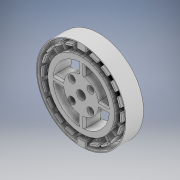
# Autodesk Inventor part: Kotač_v.2.0
Saved by Autodesk Inventor 2020 (Build 240168000, 168)
## iProperties
Created: 2020-03-09
Part Number: Kotač_v.2.0
Material: Generic
Document SubType Name: Modeling
Designer: Jadran Jelčić
Density: 1 g/cm^3
Appearance: Default
Author: Jadran Jelčić
Autodesk Inventor part; units mm, degrees
ref_plane "YZ Plane" through (0, 0, 0) normal (1, 0, 0) x (0, 1, 0)
ref_plane "XZ Plane" through (0, 0, 0) normal (0, 1, 0) x (-1, 0, 0)
ref_plane "XY Plane" through (0, 0, 0) normal (0, 0, 1) x (1, 0, 0)
sketch "Sketch1" plane through (0, 0, 0) normal (0, 0, 1) x (1, 0, 0)
  circle A0 centre (0, 0) radius 19
  circle A1 centre (0, 0) radius 10
  circle A2 centre (0, 0) radius 2.5
  line L0 (0, 0) -> (-75, 0)
  line L1 (0, 0) -> (-7.5, 0)
  circle A3 centre (-7.5, 0) radius 2
  circle A4 centre (0, -7.5) radius 2
  circle A5 centre (7.5, 0) radius 2
  circle A6 centre (0, 7.5) radius 2
  circle A7 centre (0, 0) radius 16
  line L2 (-9.8406, 1.7786) -> (-15.9008, 1.7786)
  line L3 (-9.8331, -1.8195) -> (-15.8962, -1.8195)
  line L4 (-1.7786, -9.8406) -> (-1.7786, -15.9008)
  line L5 (1.8195, -9.8331) -> (1.8195, -15.8962)
  line L6 (9.8406, -1.7786) -> (15.9008, -1.7786)
  line L7 (9.8331, 1.8195) -> (15.8962, 1.8195)
  line L8 (1.7786, 9.8406) -> (1.7786, 15.9008)
  line L9 (-1.8195, 9.8331) -> (-1.8195, 15.8962)
  line L10 (0, -7.5) -> (-7.5, 0)
  line L11 (0, 0) -> (-9.2351, -9.2351)
  line L12 (0, 0) -> (13.0604, 0) construction
  circle A8 centre (-5.3039, -5.3039) radius 2
  circle A9 centre (5.3039, -5.3039) radius 2
  circle A10 centre (5.3039, 5.3039) radius 2
  circle A11 centre (-5.3039, 5.3039) radius 2
  point P0 (-1.7786, -9.8406)
  point P1 (-1.7786, -15.9008)
  point P2 (1.8195, -15.8962)
  point P3 (1.8195, -9.8331)
  point P4 (9.8406, -1.7786)
  point P5 (15.8962, 1.8195)
  point P6 (9.8331, 1.8195)
  point P7 (1.7786, 9.8406)
  point P8 (-1.8195, 15.8962)
  point P9 (-1.8195, 9.8331)
  dimension "d0" = 38
  dimension "d1" = 20
  dimension "d2" = 5
  dimension "d5" = 4
  dimension "d8" = 360
  dimension "d12" = 360
  dimension "d23" = 32
  dimension "d31" = 135
  dimension "d32" = 4
  dimension "d35" = 360
  constraints: 26 end point, 12 centre point, 5 coincident, 4 point on circle, 2 horizontal, 2 parallel, 2 point on line, 1 equal length, 43 other
  measures "d0" diameter of A0
  measures "d1" diameter of A1
  measures "d2" diameter of A2
  measures "d5" diameter of A3
  measures "d23" diameter of A7
  measures "d31" angle of L11 L12
  measures "d32" diameter of A8
extrude "Extrusion1" add sketch "Sketch1" along normal blind 10 contours A0 | A1 L11 A8 A2 L0 A3 | A1 L7 A7 L6 | A1 L9 A7 L8 | L5 A7 L4 A1 | A1 L0 A7 L2 | A1 L0 A3 L10 L11 A8 | A1 L3 A7 L0 | A8 L11 | L11 A8 | L0 A2 L11 L10 A3 | A9 | A10 | A11
sketch "Sketch2" plane through (0, 0, 10) normal (0, 0, 1) x (1, 0, 0)
  circle A0 centre (0, 0) radius 2.5 projected
  circle A1 centre (0, 0) radius 19 projected
  line L0 (-19, 0) -> (-23, 0)
  line L1 (-23, 0) -> (-23, 0.991)
  line L2 (-23, 0.991) -> (-18.9741, 0.991)
  line L3 (-23, 0.991) -> (-23, 2.3883)
  line L4 (-23, 2.3883) -> (-22, 2.3883)
  line L5 (-22, 2.3883) -> (-22, 0.991)
  line L6 (-23, 0) -> (-23, -0.991)
  line L7 (-23, -0.991) -> (-18.9741, -0.991)
  line L8 (-23, -0.991) -> (-23, -2.3883)
  line L9 (-23, -2.3883) -> (-22, -2.3883)
  line L10 (-22, -2.3883) -> (-22, -0.991)
  point P0 (-18.9741, -0.991)
  dimension "d18" = 1
  dimension "d19" = 4
  constraints: 22 end point, 5 symmetric about line, 4 perpendicular, 2 point on circle, 2 point on line, 1 horizontal, 1 vertical
  measures "d18" distance between parallel lines of L5 L3
  measures "d19" distance from line of L0.start L1
extrude "Extrusion7" add sketch "Sketch2" against normal blind 10 contours A1 L0 L1 L2 | L7 L6 L0 A1 | L2 L3 L4 L5 | L10 L9 L8 L7
pattern_circular "Circular Pattern2" count 20 over 360 about axis through (0, 0, 0) along (0, 0, 1) of "Extrusion7"
sketch "Sketch4" plane through (0, 0, 10) normal (0, 0, 1) x (1, 0, 0)
  line L0 (0, 0) -> (-2.7237, 0)
  line L1 (2.3883, -22) -> (2.3883, -23) projected
  line L2 (2.3883, -23) -> (-2.3771, -23)
  line L3 (-2.3771, -23) -> (-2.3771, -25)
  line L4 (-2.3771, -25) -> (2.3883, -25)
  line L5 (2.3883, -25) -> (2.3883, -23)
  line L6 (2.3883, 22) -> (2.3883, 23)
  line L7 (2.3883, 23) -> (-2.3771, 23)
  line L8 (-2.3771, 23) -> (-2.3771, 25)
  line L9 (-2.3771, 25) -> (2.3883, 25)
  line L10 (2.3883, 25) -> (2.3883, 23)
  dimension "d52" = 2
  constraints: 20 end point, 5 symmetric about line, 2 horizontal, 2 parallel, 1 perpendicular
  measures "d52" distance of L3.end L2.end
extrude "Extrusion8" add sketch "Sketch4" against normal blind 1
sketch "Sketch5" plane through (0, 0, 10) normal (0, 0, 1) x (1, 0, 0)
  circle A0 centre (0, 0) radius 2.5 projected
  circle A1 centre (0, 0) radius 25
  circle A2 centre (0, 0) radius 25.5
  dimension "d27" = 50
  dimension "d28" = 51
  constraints: 2 centre point, 2 coincident
  measures "d27" diameter of A1
  measures "d28" diameter of A2
extrude "Extrusion4" add sketch "Sketch5" against normal blind 10 contours A2
sketch "Sketch8" plane through (0, 0, 10) normal (0, 0, 1) x (1, 0, 0)
  line L0 (-0.991, 18.9741) -> (-0.991, 22) projected
  line L1 (0.991, 22) -> (0.991, 18.9741) projected
  line L2 (-0.991, 22) -> (0.991, 22)
  line L3 (0.991, 22) -> (0.991, 18.9741)
  line L4 (0.991, 18.9741) -> (-0.991, 18.9741)
  line L5 (-0.991, 18.9741) -> (-0.991, 22)
  arc A0 (4.9208, 18.3517) -> (0.991, 18.9741) centre (0, 0) ccw projected
  line L6 (-6.8058, 17.7392) -> (-7.7409, 20.617)
  line L7 (-7.7409, 20.617) -> (-5.8559, 21.2295)
  line L8 (-5.8559, 21.2295) -> (-4.9208, 18.3517)
  line L9 (-4.9208, 18.3517) -> (-6.8058, 17.7392)
  line L10 (-11.9545, 14.7679) -> (-13.733, 17.2159)
  line L11 (-13.733, 17.2159) -> (-12.1295, 18.3809)
  line L12 (-12.1295, 18.3809) -> (-10.351, 15.9329)
  line L13 (-10.351, 15.9329) -> (-11.9545, 14.7679)
  line L14 (-15.9329, 10.351) -> (-18.3809, 12.1295)
  line L15 (-18.3809, 12.1295) -> (-17.2159, 13.733)
  line L16 (-17.2159, 13.733) -> (-14.7679, 11.9545)
  line L17 (-14.7679, 11.9545) -> (-15.9329, 10.351)
  line L18 (-18.3517, 4.9208) -> (-21.2295, 5.8559)
  line L19 (-21.2295, 5.8559) -> (-20.617, 7.7409)
  line L20 (-20.617, 7.7409) -> (-17.7392, 6.8058)
  line L21 (-17.7392, 6.8058) -> (-18.3517, 4.9208)
  line L22 (-18.9741, -0.991) -> (-22, -0.991)
  line L23 (-22, -0.991) -> (-22, 0.991)
  line L24 (-22, 0.991) -> (-18.9741, 0.991)
  line L25 (-18.9741, 0.991) -> (-18.9741, -0.991)
  line L26 (-17.7392, -6.8058) -> (-20.617, -7.7409)
  line L27 (-20.617, -7.7409) -> (-21.2295, -5.8559)
  line L28 (-21.2295, -5.8559) -> (-18.3517, -4.9208)
  line L29 (-18.3517, -4.9208) -> (-17.7392, -6.8058)
  line L30 (-14.7679, -11.9545) -> (-17.2159, -13.733)
  line L31 (-17.2159, -13.733) -> (-18.3809, -12.1295)
  line L32 (-18.3809, -12.1295) -> (-15.9329, -10.351)
  line L33 (-15.9329, -10.351) -> (-14.7679, -11.9545)
  line L34 (-10.351, -15.9329) -> (-12.1295, -18.3809)
  line L35 (-12.1295, -18.3809) -> (-13.733, -17.2159)
  line L36 (-13.733, -17.2159) -> (-11.9545, -14.7679)
  line L37 (-11.9545, -14.7679) -> (-10.351, -15.9329)
  line L38 (-4.9208, -18.3517) -> (-5.8559, -21.2295)
  line L39 (-5.8559, -21.2295) -> (-7.7409, -20.617)
  line L40 (-7.7409, -20.617) -> (-6.8058, -17.7392)
  line L41 (-6.8058, -17.7392) -> (-4.9208, -18.3517)
  line L42 (0.991, -18.9741) -> (0.991, -22)
  line L43 (0.991, -22) -> (-0.991, -22)
  line L44 (-0.991, -22) -> (-0.991, -18.9741)
  line L45 (-0.991, -18.9741) -> (0.991, -18.9741)
  line L46 (6.8058, -17.7392) -> (7.7409, -20.617)
  line L47 (7.7409, -20.617) -> (5.8559, -21.2295)
  line L48 (5.8559, -21.2295) -> (4.9208, -18.3517)
  line L49 (4.9208, -18.3517) -> (6.8058, -17.7392)
  line L50 (11.9545, -14.7679) -> (13.733, -17.2159)
  line L51 (13.733, -17.2159) -> (12.1295, -18.3809)
  line L52 (12.1295, -18.3809) -> (10.351, -15.9329)
  line L53 (10.351, -15.9329) -> (11.9545, -14.7679)
  line L54 (15.9329, -10.351) -> (18.3809, -12.1295)
  line L55 (18.3809, -12.1295) -> (17.2159, -13.733)
  line L56 (17.2159, -13.733) -> (14.7679, -11.9545)
  line L57 (14.7679, -11.9545) -> (15.9329, -10.351)
  line L58 (18.3517, -4.9208) -> (21.2295, -5.8559)
  line L59 (21.2295, -5.8559) -> (20.617, -7.7409)
  line L60 (20.617, -7.7409) -> (17.7392, -6.8058)
  line L61 (17.7392, -6.8058) -> (18.3517, -4.9208)
  line L62 (18.9741, 0.991) -> (22, 0.991)
  line L63 (22, 0.991) -> (22, -0.991)
  line L64 (22, -0.991) -> (18.9741, -0.991)
  line L65 (18.9741, -0.991) -> (18.9741, 0.991)
  line L66 (17.7392, 6.8058) -> (20.617, 7.7409)
  line L67 (20.617, 7.7409) -> (21.2295, 5.8559)
  line L68 (21.2295, 5.8559) -> (18.3517, 4.9208)
  line L69 (18.3517, 4.9208) -> (17.7392, 6.8058)
  line L70 (14.7679, 11.9545) -> (17.2159, 13.733)
  line L71 (17.2159, 13.733) -> (18.3809, 12.1295)
  line L72 (18.3809, 12.1295) -> (15.9329, 10.351)
  line L73 (15.9329, 10.351) -> (14.7679, 11.9545)
  line L74 (10.351, 15.9329) -> (12.1295, 18.3809)
  line L75 (12.1295, 18.3809) -> (13.733, 17.2159)
  line L76 (13.733, 17.2159) -> (11.9545, 14.7679)
  line L77 (11.9545, 14.7679) -> (10.351, 15.9329)
  line L78 (4.9208, 18.3517) -> (5.8559, 21.2295)
  line L79 (5.8559, 21.2295) -> (7.7409, 20.617)
  line L80 (7.7409, 20.617) -> (6.8058, 17.7392)
  line L81 (6.8058, 17.7392) -> (4.9208, 18.3517)
  dimension "d57" = 360
  constraints: 160 end point, 2 parallel, 1 horizontal, 1 perpendicular, 161 other
extrude "Extrusion9" cut sketch "Sketch8" against normal blind 2.5
sketch "Sketch9" plane through (0, 0, 0) normal (0, 0, -1) x (-1, 0, 0)
  arc A0 (-18.3517, 4.9208) -> (-18.9741, 0.991) centre (0, 0) ccw projected
  line L0 (-22, -2.3883) -> (-22, -0.991) projected
  line L1 (-18.9741, 0.991) -> (-22, 0.991) projected
  line L2 (-22, -0.991) -> (-18.9741, -0.991)
  line L3 (-18.9741, -0.991) -> (-18.9741, 0.991)
  line L4 (-18.9741, 0.991) -> (-22, 0.991)
  line L5 (-22, 0.991) -> (-22, -0.991)
  line L6 (-21.2295, -5.8559) -> (-20.617, -7.7409)
  line L7 (-20.617, -7.7409) -> (-17.7392, -6.8058)
  line L8 (-18.3517, -4.9208) -> (-21.2295, -5.8559)
  line L9 (-17.7392, -6.8058) -> (-18.3517, -4.9208)
  line L10 (-18.3809, -12.1295) -> (-17.2159, -13.733)
  line L11 (-17.2159, -13.733) -> (-14.7679, -11.9545)
  line L12 (-15.9329, -10.351) -> (-18.3809, -12.1295)
  line L13 (-14.7679, -11.9545) -> (-15.9329, -10.351)
  line L14 (-13.733, -17.2159) -> (-12.1295, -18.3809)
  line L15 (-12.1295, -18.3809) -> (-10.351, -15.9329)
  line L16 (-11.9545, -14.7679) -> (-13.733, -17.2159)
  line L17 (-10.351, -15.9329) -> (-11.9545, -14.7679)
  line L18 (-7.7409, -20.617) -> (-5.8559, -21.2295)
  line L19 (-5.8559, -21.2295) -> (-4.9208, -18.3517)
  line L20 (-6.8058, -17.7392) -> (-7.7409, -20.617)
  line L21 (-4.9208, -18.3517) -> (-6.8058, -17.7392)
  line L22 (-0.991, -22) -> (0.991, -22)
  line L23 (0.991, -22) -> (0.991, -18.9741)
  line L24 (-0.991, -18.9741) -> (-0.991, -22)
  line L25 (0.991, -18.9741) -> (-0.991, -18.9741)
  line L26 (5.8559, -21.2295) -> (7.7409, -20.617)
  line L27 (7.7409, -20.617) -> (6.8058, -17.7392)
  line L28 (4.9208, -18.3517) -> (5.8559, -21.2295)
  line L29 (6.8058, -17.7392) -> (4.9208, -18.3517)
  line L30 (12.1295, -18.3809) -> (13.733, -17.2159)
  line L31 (13.733, -17.2159) -> (11.9545, -14.7679)
  line L32 (10.351, -15.9329) -> (12.1295, -18.3809)
  line L33 (11.9545, -14.7679) -> (10.351, -15.9329)
  line L34 (17.2159, -13.733) -> (18.3809, -12.1295)
  line L35 (18.3809, -12.1295) -> (15.9329, -10.351)
  line L36 (14.7679, -11.9545) -> (17.2159, -13.733)
  line L37 (15.9329, -10.351) -> (14.7679, -11.9545)
  line L38 (20.617, -7.7409) -> (21.2295, -5.8559)
  line L39 (21.2295, -5.8559) -> (18.3517, -4.9208)
  line L40 (17.7392, -6.8058) -> (20.617, -7.7409)
  line L41 (18.3517, -4.9208) -> (17.7392, -6.8058)
  line L42 (22, -0.991) -> (22, 0.991)
  line L43 (22, 0.991) -> (18.9741, 0.991)
  line L44 (18.9741, -0.991) -> (22, -0.991)
  line L45 (18.9741, 0.991) -> (18.9741, -0.991)
  line L46 (21.2295, 5.8559) -> (20.617, 7.7409)
  line L47 (20.617, 7.7409) -> (17.7392, 6.8058)
  line L48 (18.3517, 4.9208) -> (21.2295, 5.8559)
  line L49 (17.7392, 6.8058) -> (18.3517, 4.9208)
  line L50 (18.3809, 12.1295) -> (17.2159, 13.733)
  line L51 (17.2159, 13.733) -> (14.7679, 11.9545)
  line L52 (15.9329, 10.351) -> (18.3809, 12.1295)
  line L53 (14.7679, 11.9545) -> (15.9329, 10.351)
  line L54 (13.733, 17.2159) -> (12.1295, 18.3809)
  line L55 (12.1295, 18.3809) -> (10.351, 15.9329)
  line L56 (11.9545, 14.7679) -> (13.733, 17.2159)
  line L57 (10.351, 15.9329) -> (11.9545, 14.7679)
  line L58 (7.7409, 20.617) -> (5.8559, 21.2295)
  line L59 (5.8559, 21.2295) -> (4.9208, 18.3517)
  line L60 (6.8058, 17.7392) -> (7.7409, 20.617)
  line L61 (4.9208, 18.3517) -> (6.8058, 17.7392)
  line L62 (0.991, 22) -> (-0.991, 22)
  line L63 (-0.991, 22) -> (-0.991, 18.9741)
  line L64 (0.991, 18.9741) -> (0.991, 22)
  line L65 (-0.991, 18.9741) -> (0.991, 18.9741)
  line L66 (-5.8559, 21.2295) -> (-7.7409, 20.617)
  line L67 (-7.7409, 20.617) -> (-6.8058, 17.7392)
  line L68 (-4.9208, 18.3517) -> (-5.8559, 21.2295)
  line L69 (-6.8058, 17.7392) -> (-4.9208, 18.3517)
  line L70 (-12.1295, 18.3809) -> (-13.733, 17.2159)
  line L71 (-13.733, 17.2159) -> (-11.9545, 14.7679)
  line L72 (-10.351, 15.9329) -> (-12.1295, 18.3809)
  line L73 (-11.9545, 14.7679) -> (-10.351, 15.9329)
  line L74 (-17.2159, 13.733) -> (-18.3809, 12.1295)
  line L75 (-18.3809, 12.1295) -> (-15.9329, 10.351)
  line L76 (-14.7679, 11.9545) -> (-17.2159, 13.733)
  line L77 (-15.9329, 10.351) -> (-14.7679, 11.9545)
  line L78 (-20.617, 7.7409) -> (-21.2295, 5.8559)
  line L79 (-21.2295, 5.8559) -> (-18.3517, 4.9208)
  line L80 (-17.7392, 6.8058) -> (-20.617, 7.7409)
  line L81 (-18.3517, 4.9208) -> (-17.7392, 6.8058)
  point P0 (-21.2295, -5.8559)
  point P1 (-18.3809, -12.1295)
  point P2 (-13.733, -17.2159)
  point P3 (-7.7409, -20.617)
  point P4 (-0.991, -22)
  point P5 (5.8559, -21.2295)
  point P6 (12.1295, -18.3809)
  point P7 (17.2159, -13.733)
  point P8 (20.617, -7.7409)
  point P9 (22, -0.991)
  point P10 (21.2295, 5.8559)
  point P11 (18.3809, 12.1295)
  point P12 (13.733, 17.2159)
  point P13 (7.7409, 20.617)
  point P14 (0.991, 22)
  point P15 (-5.8559, 21.2295)
  point P16 (-12.1295, 18.3809)
  point P17 (-17.2159, 13.733)
  point P18 (-20.617, 7.7409)
  dimension "d63" = 360
  constraints: 160 end point, 2 parallel, 1 horizontal, 1 perpendicular, 181 other
extrude "Extrusion10" cut sketch "Sketch9" against normal blind 2.5
sketch "Sketch6" plane through (0, 0, 10) normal (0, 0, 1) x (1, 0, 0)
  circle A0 centre (0, 0) radius 2.5 projected
  circle A1 centre (0, 0) radius 7.5
  circle A2 centre (5.3033, -5.3033) radius 2
  circle A3 centre (5.3033, 5.3033) radius 2
  circle A4 centre (-5.3033, 5.3033) radius 2
  circle A5 centre (-5.3033, -5.3033) radius 2
  dimension "d37" = 15
  dimension "d38" = 4
  dimension "d41" = 360
  constraints: 4 centre point, 1 coincident, 12 other
  measures "d38" diameter of A2
extrude "Extrusion5" cut sketch "Sketch6" against normal blind 15 contours A3 A1 | A1 A3 | A2 A1 | A1 A2 | A4 A1 | A1 A4 | A5 A1 | A1 A5
sketch "Sketch7" plane through (0, 0, 10) normal (0, 0, 1) x (1, 0, 0)
  circle A0 centre (-7.5, 0) radius 2 projected
  circle A1 centre (0, -7.5) radius 2 projected
  circle A2 centre (7.5, 0) radius 2 projected
  circle A3 centre (0, 7.5) radius 2 projected
  circle A4 centre (-7.5, 0) radius 2
  circle A5 centre (0, -7.5) radius 2
  circle A6 centre (7.5, 0) radius 2
  circle A7 centre (0, 7.5) radius 2
  point P0 (0, 0)
  constraints: 4 centre point, 4 coincident, 4 concentric
extrude "Extrusion6" add sketch "Sketch7" against normal blind 10
fillet "Fillet1" radius 1 16 edges at (-1.7786, -12.8707, 0) (1.8195, -12.8646, 0) (-1.7786, -12.8707, 10) (1.8195, -12.8646, 10) (12.8707, -1.7786, 10) (12.8646, 1.8195, 10) (12.8646, 1.8195, 0) (12.8707, -1.7786, 0) (1.7786, 12.8707, 0) (-1.8195, 12.8646, 0) (-12.8707, 1.7786, 0) (-12.8646, -1.8195, 0) (1.7786, 12.8707, 10) (-1.8195, 12.8646, 10) (-12.8646, -1.8195, 10) (-12.8707, 1.7786, 10)
sketch "Sketch10" plane through (0, 0, 7.5) normal (0, 0, 1) x (1, 0, 0)
  point P0 (0, 0)
body "Solid1"
